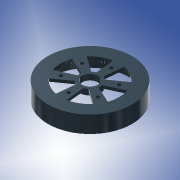
# Autodesk Inventor part: Spur Gear1
Saved by Autodesk Inventor 2017 SP1 (Build 210196100, 196)
## iProperties
Created: 2017-07-05
Part Number: Spur Gear1
Material: ABS Plastic
Document SubType Name: Modeling
Designer: zallen
Categories: <?xml version="1.0" encoding="UTF-16"?> <MemberInstance><Categories><FamilyTemplate><FamilyTemplateParameter ValueType="xs:double" Id="1" ObjectReferenceKey="da_z" ObjectType="kUserParameterObject"/><FamilyTemplateParameter ValueType="xs:double" Id="2" ObjectReferenceKey="da_b" ObjectType="kUserParameterObject"/><FamilyTemplateParameter ValueType="xs:double" Id="3" ObjectReferenceKey="da_beta" ObjectType="kUserParameterObject"/><FamilyTemplateParameter ValueType="xs:double" Id="4" ObjectReferenceKey="da_da" ObjectType="kUserParameterObject"/><FamilyTemplateParameter ValueType="xs:double" Id="5" ObjectReferenceKey="da_aw" ObjectType="kUserParameterObject"/><FamilyTemplateParameter ValueType="xs:string" Id="6" ObjectReferenceKey="EAIAABAAAACIAQAAAAAAAIAAAAAAAAAA" ObjectType="83910656" SubObjectId="SurfaceGeometry"/></FamilyTemplate><ParamToTemplateMap><ParamToTemplate CategoryParameter="//CategoryParameter[@InternalName='046C89C9-8512-4d59-83FE-43B91F4F132A']" TemplateParameter="1"/><ParamToTemplate CategoryParameter="//CategoryParameter[@InternalName='2552DF32-E462-4b46-AEBF-C6C7768E72AC']" TemplateParameter="2"/><ParamToTemplate CategoryParameter="//CategoryParameter[@InternalName='C9EE641D-15FC-4fae-A226-E94C4372FDD7']" TemplateParameter="3"/><ParamToTemplate><ParamToTemplate CategoryParameter="//CategoryParameter[@InternalName='00B6519A-459B-49c7-AD84-2E56D39A5744']" ConstantValue="-0.200000"/></ParamToTemplate><ParamToTemplate><ParamToTemplate CategoryParameter="//CategoryParameter[@InternalName='04B31F0E-C7A6-4894-AA32-9629BEFACF47']" ConstantValue="1.000000"/></ParamToTemplate><ParamToTemplate><ParamToTemplate CategoryParameter="//CategoryParameter[@InternalName='43CBEC2E-7847-49e7-A936-2F7889FCB2D9']" ConstantValue="0.250000"/></ParamToTemplate><ParamToTemplate><ParamToTemplate CategoryParameter="//CategoryParameter[@InternalName='B1EFC894-105D-4ebd-86BF-FA20ED196853']" ConstantValue="0.302500"/></ParamToTemplate><ParamToTemplate><ParamToTemplate CategoryParameter="//CategoryParameter[@InternalName='51175063-3D10-4879-93E8-6246FE8B403D']" ConstantValue="2060000000.000000"/></ParamToTemplate><ParamToTemplate><ParamToTemplate CategoryParameter="//CategoryParameter[@InternalName='A3A52E27-4454-46a9-B0BD-C932399B70AF']" ConstantValue="0.300000"/></ParamToTemplate><ParamToTemplate><ParamToTemplate CategoryParameter="//CategoryParameter[@InternalName='91B76062-C214-41d9-B1B9-14D2AB99603D']" ConstantValue="0.100000"/></ParamToTemplate><ParamToTemplate><ParamToTemplate CategoryParameter="//CategoryParameter[@InternalName='374E806E-8B8A-4dda-A9AA-1039D6500AD2']" ConstantValue="10.000000"/></ParamToTemplate><ParamToTemplate><ParamToTemplate CategoryParameter="//CategoryParameter[@InternalName='2D373A89-B862-43d6-8D0B-0CBF12AB9F6C']" ConstantValue="0.174533"/></ParamToTemplate><ParamToTemplate CategoryParameter="//CategoryParameter[@InternalName='37777632-D6A2-4fac-9D53-DB8ACD95C989']" TemplateParameter="4"/><ParamToTemplate CategoryParameter="//CategoryParameter[@InternalName='FD1017F1-B727-4f7e-9707-0F86F1FF9423']" TemplateParameter="5"/><ParamToTemplate><ParamToTemplate CategoryParameter="//CategoryParameter[@InternalName='9E1B4470-B2D3-4ff1-B813-535BB4CDF51A']" ConstantValue="3520000.000000"/></ParamToTemplate><ParamToTemplate><ParamToTemplate CategoryParameter="//CategoryParameter[@InternalName='F8452263-BFF6-458c-9FB1-07C4B99E95CD']" ConstantValue="11400000.000000"/></ParamToTemplate><ParamToTemplate><ParamToTemplate CategoryParameter="//CategoryParameter[@InternalName='3E3BB259-FD49-497f-8171-6EBC954A3479']" ConstantValue="2.000000"/></ParamToTemplate><ParamToTemplate CategoryParameter="//CategoryParameter[@InternalName='27C3BAF2-7550-4e4b-AE2C-0DB134B7D9B7']" TemplateParameter="6"/></ParamToTemplateMap><Category DisplayName="Gear" InternalName="DC85795E-93AB-48d5-8EEE-5A27447B64BD" Mnemonic="Gear"><CategoryParameter DisplayName="z" InternalName="046C89C9-8512-4d59-83FE-43B91F4F132A" Mnemonic="z"/><CategoryParameter DisplayName="b" InternalName="2552DF32-E462-4b46-AEBF-C6C7768E72AC" Mnemonic="b"/><CategoryParameter DisplayName="||b|" InternalName="C9EE641D-15FC-4fae-A226-E94C4372FDD7" Mnemonic="beta"/><CategoryParameter DisplayName="x" InternalName="00B6519A-459B-49c7-AD84-2E56D39A5744" Mnemonic="x"/><CategoryParameter DisplayName="a*" InternalName="04B31F0E-C7A6-4894-AA32-9629BEFACF47" Mnemonic="a"/><CategoryParameter DisplayName="c*" InternalName="43CBEC2E-7847-49e7-A936-2F7889FCB2D9" Mnemonic="c"/><CategoryParameter DisplayName="r|.f|*" InternalName="B1EFC894-105D-4ebd-86BF-FA20ED196853" Mnemonic="rf"/><CategoryParameter DisplayName="E" InternalName="51175063-3D10-4879-93E8-6246FE8B403D" Mnemonic="E"/><CategoryParameter DisplayName="||m|" InternalName="A3A52E27-4454-46a9-B0BD-C932399B70AF" Mnemonic="mi"/><Category DisplayName="SpurGear" InternalName="26C5A22E-A91E-4dfd-A3B3-23CCAFAE1764" Mnemonic="SpurGear"><CategoryParameter DisplayName="m" InternalName="91B76062-C214-41d9-B1B9-14D2AB99603D" Mnemonic="m"/><CategoryParameter DisplayName="P" InternalName="374E806E-8B8A-4dda-A9AA-1039D6500AD2" Mnemonic="PP"/><CategoryParameter DisplayName="||a|" InternalName="2D373A89-B862-43d6-8D0B-0CBF12AB9F6C" Mnemonic="alpha"/><CategoryParameter DisplayName="d|.a|" InternalName="37777632-D6A2-4fac-9D53-DB8ACD95C989" Mnemonic="da"/><CategoryParameter DisplayName="a|.w|" InternalName="FD1017F1-B727-4f7e-9707-0F86F1FF9423" Mnemonic="aw"/><CategoryParameter DisplayName="||s||.Flim|" InternalName="9E1B4470-B2D3-4ff1-B813-535BB4CDF51A" Mnemonic="sFlim"/><CategoryParameter DisplayName="||s||.Hlim|" InternalName="F8452263-BFF6-458c-9FB1-07C4B99E95CD" Mnemonic="sHlim"/><CategoryParameter DisplayName="type" InternalName="3E3BB259-FD49-497f-8171-6EBC954A3479" Mnemonic="type"/><Category DisplayName="InternalSpurGear" InternalName="7CF704F6-14A9-42f8-93CE-E71DF57C2B55" Mnemonic="InternalSpurGear"><CategoryParameter DisplayName="PitchDiameter" InternalName="27C3BAF2-7550-4e4b-AE2C-0DB134B7D9B7" Mnemonic="IDS_PITCHDIAM"/></Category></Category></Category></Categories></MemberInstance>
Density: 1.06 g/cm^3
Appearance: CR Dark Blue
CustomPartVersion: 1
Author: zallen
Autodesk Inventor part; units mm, degrees
ref_plane "YZ Plane" through (0, 0, 0) normal (1, 0, 0) x (0, 1, 0)
ref_plane "XZ Plane" through (0, 0, 0) normal (0, 1, 0) x (-1, 0, 0)
ref_plane "XY Plane" through (0, 0, 0) normal (0, 0, 1) x (1, 0, 0)
sketch "Sketch1" plane through (0, 0, 0) normal (0, 0, 1) x (1, 0, 0)
  circle A0 centre (0, 0) radius 50.655
  dimension "d0" = 101.31
  constraints: 1 centre point
  measures "d0" diameter of A0
extrude "Extrusion1" add sketch "Sketch1" along normal blind 10
ref_plane "Work Plane2" through (0, 0, 5) normal (0, 0, 1) x (1, 0, 0)
sketch "Sketch2" plane through (0, 0, 0) normal (0, 0, -1) x (-1, 0, 0)
  circle A0 centre (0, 0) radius 50.655 projected
  circle A1 centre (0, 0) radius 44.7795
  dimension "d3" = 89.559
  constraints: 1 centre point, 1 coincident
  measures "d3" diameter of A1
surface extrude "Pitch Diameter" sketch "Sketch2" against normal through all shown no curves A1
ref_plane "Work Plane8" through (0, 0, 0) normal (0.9993908, 0.0348995, 0) x (0, 0, 1)
ref_plane "Work Plane9" through (0, 0, 0) normal (1, 0, 0) x (0, 1, 0)
spur gear teeth "Spur Gear" teeth 90 pitch diameter 90 tip diameter 88.9765 root diameter 92.1 face width 10 start plane through (0, 0, 0) normal (0, 0, -1) x (-1, 0, 0)
sketch "Sketch3" plane through (0, 0, 10) normal (0, 0, 1) x (1, 0, 0)
  circle A0 centre (0, 0) radius 50.655 projected
  circle A1 centre (0, 0) radius 41
  dimension "d53" = 82
  constraints: 1 centre point, 1 coincident
  measures "d53" diameter of A1
extrude "Extrusion2" add sketch "Sketch3" against normal blind 4
sketch "Sketch4" plane through (0, 0, 10) normal (0, 0, 1) x (1, 0, 0)
  circle A0 centre (0, 0) radius 11
  circle A1 centre (0, 0) radius 15
  dimension "d56" = 22
  dimension "d57" = 30
  constraints: 2 centre point, 2 coincident
  measures "d56" diameter of A0
  measures "d57" diameter of A1
extrude "Extrusion3" add sketch "Sketch4" against normal blind 8
sketch "Sketch5" plane through (0, 0, 10) normal (0, 0, 1) x (1, 0, 0)
  circle A0 centre (0, 0) radius 15 projected
  line L0 (-5, 14.1421) -> (-7.5, 40.3082)
  line L1 (5, 14.1421) -> (7.5, 40.3082)
  line L2 (0, 0) -> (0, 65.7553) construction
  arc A1 (5, 14.1421) -> (-5, 14.1421) centre (0, 0) ccw
  arc A2 (7.5, 40.3082) -> (-7.5, 40.3082) centre (0, 0) ccw
  circle A3 centre (0, 0) radius 41 projected
  line L3 (-14.7474, 2.7409) -> (-38.6579, 13.6589)
  arc A4 (-31.1579, 26.6493) -> (-38.6579, 13.6589) centre (0, 0) ccw
  line L4 (-9.7474, 11.4012) -> (-31.1579, 26.6493)
  arc A5 (-9.7474, 11.4012) -> (-14.7474, 2.7409) centre (0, 0) ccw
  line L5 (-9.7474, -11.4012) -> (-31.1579, -26.6493)
  arc A6 (-38.6579, -13.6589) -> (-31.1579, -26.6493) centre (0, 0) ccw
  line L6 (-14.7474, -2.7409) -> (-38.6579, -13.6589)
  arc A7 (-14.7474, -2.7409) -> (-9.7474, -11.4012) centre (0, 0) ccw
  line L7 (5, -14.1421) -> (7.5, -40.3082)
  arc A8 (-7.5, -40.3082) -> (7.5, -40.3082) centre (0, 0) ccw
  line L8 (-5, -14.1421) -> (-7.5, -40.3082)
  arc A9 (-5, -14.1421) -> (5, -14.1421) centre (0, 0) ccw
  line L9 (14.7474, -2.7409) -> (38.6579, -13.6589)
  arc A10 (31.1579, -26.6493) -> (38.6579, -13.6589) centre (0, 0) ccw
  line L10 (9.7474, -11.4012) -> (31.1579, -26.6493)
  arc A11 (9.7474, -11.4012) -> (14.7474, -2.7409) centre (0, 0) ccw
  line L11 (9.7474, 11.4012) -> (31.1579, 26.6493)
  arc A12 (38.6579, 13.6589) -> (31.1579, 26.6493) centre (0, 0) ccw
  line L12 (14.7474, 2.7409) -> (38.6579, 13.6589)
  arc A13 (14.7474, 2.7409) -> (9.7474, 11.4012) centre (0, 0) ccw
  dimension "d60" = 10
  dimension "d61" = 15
  dimension "d64" = 360
  constraints: 28 point on circle, 26 end point, 12 centre point, 2 coincident, 2 concentric, 1 vertical, 60 other
  measures "d60" distance of L1.start L0.start
  measures "d61" distance of L1.end L0.end
extrude "Extrusion4" add sketch "Sketch5" against normal blind 4 contours A0 L11 A3 L12 | L9 A3 L10 A0 | A0 L0 A2 L1 | L7 A3 L8 A0 | A0 L3 A3 L4 | L5 A3 L6 A0
sketch "Sketch6" plane through (0, 0, 10) normal (0, 0, 1) x (1, 0, 0)
  circle A0 centre (0, 30) radius 2.5
  line L0 (0, 0) -> (0, 56.091) construction
  circle A1 centre (-25.9808, 15) radius 2.5
  circle A2 centre (-25.9808, -15) radius 2.5
  circle A3 centre (0, -30) radius 2.5
  circle A4 centre (25.9808, -15) radius 2.5
  circle A5 centre (25.9808, 15) radius 2.5
  dimension "d68" = 5
  dimension "d69" = 30
  dimension "d72" = 360
  constraints: 6 centre point, 2 end point, 1 point on line, 1 vertical, 13 other
  measures "d68" diameter of A0
  measures "d69" distance of L0.start A0.centre
extrude "Extrusion5" cut sketch "Sketch6" against normal through all
sketch "Sketch7" plane through (0, 0, 10) normal (0, 0, 1) x (1, 0, 0)
  circle A0 centre (0, 0) radius 50.655 projected
  circle A1 centre (0, 0) radius 55
  dimension "d76" = 110
  constraints: 1 centre point, 1 coincident
  measures "d76" diameter of A1
extrude "Extrusion6" add sketch "Sketch7" against normal blind 4
sketch "Sketch8" plane through (0, 0, 10) normal (0, 0, 1) x (1, 0, 0)
  circle A0 centre (0, 0) radius 59
  circle A1 centre (0, 0) radius 55 projected
  dimension "d79" = 118
  constraints: 1 centre point, 1 coincident
  measures "d79" diameter of A0
extrude "Extrusion7" add sketch "Sketch8" against normal blind 23.75
equation "\"d0\" = 1.1 * da_df"
equation "\"d1\" = da_b"
equation "\"d3\" = da_dw"
equation "\"d16\" = da_aw"
equation "\"d47\" = da_aw"
equation "\"d52\" = da_aw"
equation "\"da_df\" = 92.1"
equation "\"da_b\" = 10"
equation "\"da_dw\" = 89.558963"
equation "\"da_aw\" = 22.389741"
body "Solid1"
body "Srf1"
